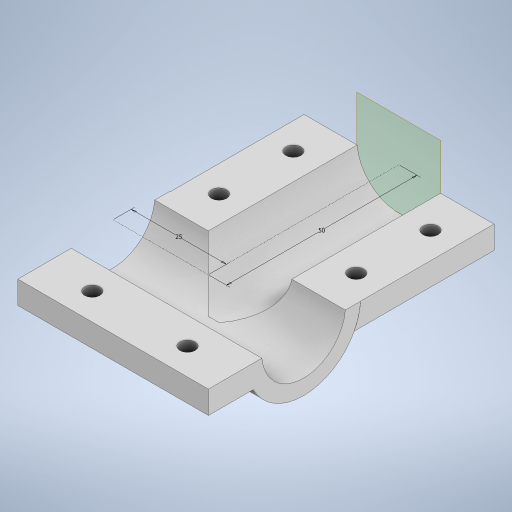
# Autodesk Inventor part: betterTconection
Saved by Autodesk Inventor 2023 (Build 270158000, 158)
## iProperties
Created: 2023-10-23
Part Number: betterTconection
Material: Generic
Document SubType Name: Modeling
Designer: Nikita
Density: 1 g/cm^3
Appearance: Default
Author: Nikita
Autodesk Inventor part; units mm, degrees
ref_plane "YZ Plane" through (0, 0, 0) normal (1, 0, 0) x (0, 1, 0)
ref_plane "XZ Plane" through (0, 0, 0) normal (0, 1, 0) x (-1, 0, 0)
ref_plane "XY Plane" through (0, 0, 0) normal (0, 0, 1) x (1, 0, 0)
sketch "Sketch1" plane through (0, 0, 0) normal (1, 0, 0) x (0, 1, 0)
  arc A0 (-1, 14.96663) -> (0, -15) centre (0, 0) ccw
  arc A1 (-1, 10.954451) -> (0, -11) centre (0, 0) ccw
  line L0 (0, 15) -> (0, -15)
  line L1 (-1, 14.96663) -> (-1, 10.954451)
  point P0 (0, 11.5)
  dimension "d0" = 30
  dimension "d1" = 22
  constraints: 4 end point, 4 point on circle, 2 centre point, 2 coincident, 2 point on line, 2 vertical
  measures "d0" diameter of A0
  measures "d1" diameter of A1
extrude "Extrusion1" add sketch "Sketch1" along normal blind 50
sketch "Sketch2" plane through (50, 0, 0) normal (1, 0, 0) x (0, 0, -1)
  line L0 (-10.954451, -1) -> (-14.96663, -1)
  line L1 (-14.96663, -1) -> (-24.96663, -1)
  line L2 (-24.96663, -1) -> (-24.96663, -7)
  line L3 (-24.96663, -7) -> (-13.211534, -7)
  arc A0 (-14.96663, -1) -> (15, 0) centre (0, 0) ccw
  line L4 (-14.96663, -1) -> (-13.211534, -7)
  point P0 (-13.266499, -7)
  dimension "d5" = 10
  dimension "d6" = 6
  constraints: 8 end point, 2 perpendicular, 1 horizontal
  measures "d5" distance of L0.end L1.end
  measures "d6" distance of L1.end L2.end
extrude "Extrusion2" add sketch "Sketch2" against normal blind 50 contours A0 L3 L2 L1
sketch "Sketch3" plane through (0, 0, 0) normal (0, 1, 0) x (-1, 0, 0)
  line L0 (0, 0) -> (-25, 0) construction
  line L1 (-25, 0) -> (-25, -50) construction
  dimension "d9" = 25
  dimension "d10" = 50
  constraints: 4 end point, 1 horizontal, 1 perpendicular
  measures "d9" distance of L0.start L0.end
  measures "d10" distance of L0.end L1.end
ref_plane "Work Plane1" through (25, 0, -50) normal (0, 0, -1) x (-1, 0, 0)
sketch "Sketch4" plane through (25, 0, -50) normal (0, 0, -1) x (-1, 0, 0)
  line L0 (25, 0) -> (-25, 0)
  arc A0 (-10.954451, -1) -> (10.954451, -1) centre (0, 0) ccw
  arc A1 (-14.96663, -1) -> (14.96663, -1) centre (0, 0) ccw
  line L1 (25, -1) -> (-25, -1)
  line L2 (-14.96663, -1) -> (14.96663, -1)
  point P0 (-10.954451, -1)
  point P1 (10.954451, -1)
  dimension "d11" = 22
  dimension "d12" = 30
  constraints: 4 point on circle, 4 point on line, 2 centre point, 2 end point, 1 coincident, 1 midpoint
  measures "d11" diameter of A0
  measures "d12" diameter of A1
extrude "Extrusion3" add sketch "Sketch4" against normal up to next contours A0 L1 A1
sketch "Sketch5" plane through (25, 0, -50) normal (0, 0, -1) x (-1, 0, 0)
  arc A0 (-10.954451, -1) -> (10.954451, -1) centre (0, 0) ccw
  circle A1 centre (0, 0) radius 11
  line L0 (25, -1) -> (-25, -1)
  line L1 (14.854796, -1) -> (24.854796, -1)
  arc A2 (-14.96663, -1) -> (0, -15) centre (0, 0) ccw
  line L2 (-14.96663, -1) -> (-24.96663, -1)
  line L3 (-24.96663, -1) -> (-24.96663, -7)
  line L4 (-24.96663, -7) -> (24.854796, -7)
  line L5 (24.854796, -7) -> (24.854796, -1)
  line L6 (-24.96663, -1) -> (24.854796, -1)
  point P0 (25, 0)
  point P1 (-13.266499, -7)
  point P2 (8.485281, -7)
  dimension "d15" = 10
  dimension "d16" = 10
  dimension "d17" = 6
  constraints: 12 end point, 3 point on line, 2 perpendicular, 1 collinear, 1 parallel, 3 other
  measures "d15" distance of L1.start L1.end
  measures "d16" distance of L2.start L2.end
  measures "d17" distance of L2.end L3.end
extrude "Extrusion4" add sketch "Sketch5" against normal blind 38.302 contours L0 L5 L4 A0 | A2 L4 L3 L0
sketch "Sketch6" plane through (25, 0, -50) normal (0, 0, -1) x (-1, 0, 0)
  line L0 (25, 0) -> (-25, 0)
  arc A0 (-10.954451, -1) -> (10.954451, -1) centre (0, 0) ccw
  circle A1 centre (0, 0) radius 11
  point P0 (-11, 0)
  point P1 (-10.954451, -1)
  point P2 (11, 0)
  constraints: 1 midpoint, 3 other
extrude "Extrusion5" cut sketch "Sketch6" against normal blind 48.552 contours A1 A0 L0
sketch "Sketch7" plane through (50, 0, -11) normal (0, 1, 0) x (1, 0, 0)
  line L0 (1.146492, -0.964321) -> (-15.803609, -0.964321)
  line L1 (-15.803609, -0.964321) -> (-15.803609, 5.725768)
  line L2 (-15.803609, 5.725768) -> (1.146492, 5.725768)
  line L3 (1.146492, 5.725768) -> (1.146492, -0.964321)
  line L4 (-26.448, -9.552) -> (-36, 0)
  line L5 (-34.667708, -1.332292) -> (-52.233675, -1.332292)
  line L6 (-52.233675, -1.332292) -> (-52.233675, 5.725768)
  line L7 (-52.233675, 5.725768) -> (-34.667708, 5.725768)
  line L8 (-34.667708, 5.725768) -> (-34.667708, -1.332292)
  point P0 (-50, -11)
  constraints: 16 end point, 4 parallel, 2 horizontal, 2 perpendicular, 1 point on line
extrude "Extrusion6" cut sketch "Sketch7" against normal blind 1
sketch "Sketch8" plane through (35.954451, -1, -10.954451) normal (0, 1, 0) x (1, 0, 0)
  line L0 (0, 39.045549) -> (14.012178, 39.045549)
  line L1 (0, 0) -> (-9.506451, -9.506451)
  line L2 (14.012178, 39.045549) -> (14.012178, 4.012178)
  line L3 (0.045549, 19.522774) -> (14.189279, 0.045549) construction
  circle A0 centre (7.117414, 9.784162) radius 2
  line L4 (0.045549, 19.522774) -> (14.012178, 39.045549) construction
  line L5 (0.045549, 19.522774) -> (-21.938424, 19.522774) construction
  line L6 (-21.938424, 19.522774) -> (-35.954451, 39.045549) construction
  line L7 (2.312048, 39.045549) -> (-24.22095, 39.045549) construction
  line L8 (-21.938424, 39.045549) -> (-35.809247, 19.522774) construction
  line L9 (-35.809247, 39.045549) -> (-35.809247, 2.312048) construction
  line L10 (7.117414, 9.784162) -> (-28.873836, 9.784162) construction
  line L11 (-28.873836, 9.784162) -> (-28.873836, 29.284162) construction
  line L12 (-28.873836, 29.284162) -> (7.117414, 29.284162) construction
  line L13 (7.117414, 29.284162) -> (7.117414, 9.784162) construction
  circle A1 centre (-28.873836, 9.784162) radius 2
  circle A2 centre (7.117414, 29.284162) radius 2
  circle A3 centre (-28.873836, 29.284162) radius 2
  line L14 (-35.954451, -21.908902) -> (14.045549, -21.908902) construction
  line L15 (-10.954451, -21.908902) -> (-35.954451, -35.954451) construction
  line L16 (-35.954451, -21.908902) -> (-35.954451, -35.921081)
  line L17 (-10.954451, -35.921081) -> (14.045549, -21.908902) construction
  line L18 (14.045549, -35.921081) -> (-35.954451, -35.921081) construction
  line L19 (14.045549, -35.921081) -> (-10.954451, -21.908902) construction
  circle A4 centre (1.545549, -28.914991) radius 2
  circle A5 centre (-23.454451, -28.914991) radius 2
  point P0 (-35.954451, -10.954451)
  dimension "d24" = 4
  dimension "d25" = 4
  dimension "d26" = 4
  dimension "d27" = 4
  dimension "d28" = 4
  dimension "d29" = 4
  constraints: 24 end point, 6 centre point, 4 midpoint, 3 coincident, 2 horizontal, 2 parallel, 2 point on line, 1 perpendicular
  measures "d24" diameter of A0
  measures "d25" diameter of A1
  measures "d26" diameter of A2
  measures "d27" diameter of A3
  measures "d28" diameter of A4
  measures "d29" diameter of A5
extrude "Extrusion7" cut sketch "Sketch8" against normal blind 48.552
body "Solid1"
